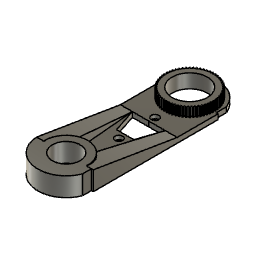
upperupperarm v1 (Autodesk Fusion 360 design; units mm, degrees)
Autodesk Fusion 360 part; units mm, degrees
sketch "lower_upper_sketch" plane through (0, 0, 0) normal (0, 0, 1) x (1, 0, 0)
  line L0 (-4.5, 9.5706) -> (-4.4999, -10)
  line L1 (0, 35.45) -> (-12.8784, 35.3615)
  circle A0 centre (0, 40.45) radius 1.75
  line L2 (0.0001, 16.7501) -> (-6.8648, 16.738)
  line L3 (0.0001, 16.7501) -> (6.9, 16.7501)
  line L4 (-4.4999, -10) -> (4.5001, -10)
  arc A1 (-4.7617, 10.2248) -> (4.7581, 10.2136) centre (0, 11.75) ccw
  arc A2 (-0.0001, 35.45) -> (0, 35.45) centre (0, 40.45) ccw
  line L5 (4.5001, -10) -> (4.5, 9.5706)
  circle A3 centre (0, 68.7017) radius 14
  line L6 (21.4115, 61.7879) -> (4.7581, 10.2136)
  circle A4 centre (0, 11.75) radius 1.75
  arc A5 (0, 45.45) -> (0, 45.45) centre (0, 67.95) ccw
  arc A6 (21.4115, 61.7879) -> (-21.4114, 61.7879) centre (0, 68.7017) ccw
  line L7 (-21.4114, 61.7879) -> (-4.7514, 10.193)
  line L8 (0, 35.45) -> (12.8942, 35.4107)
  line L9 (-4.7555, 10.2057) -> (-4.7555, 10.2055)
  circle A7 centre (50, 40.45) radius 1.75
  arc A8 (50, 45.45) -> (50.0001, 45.45) centre (50, 67.95) ccw
  circle A9 centre (50, 11.75) radius 1.75
  line L10 (50, 35.45) -> (36.9725, 35.45)
  arc A10 (72.5, 67.95) -> (29, 76.0277) centre (50, 67.95) ccw
  line L11 (50, 35.45) -> (63.0276, 35.45)
  circle A11 centre (50, 67.95) radius 14
  line L12 (50.0001, 16.7501) -> (43.1001, 16.7501)
  arc A12 (49.9999, 35.45) -> (50, 35.45) centre (50, 40.45) ccw
  line L13 (50.0001, 16.7501) -> (56.9, 16.7501)
  line L14 (50, 90.45) -> (50, -52.55) construction
  line L15 (27.5, 67.95) -> (27.5, -30.05)
  line L16 (72.5, 67.95) -> (72.5, -30.05)
  line L17 (63.0276, 35.45) -> (56.9, 16.7501)
  line L18 (36.9725, 35.45) -> (43.1001, 16.7501)
  circle A13 centre (50, -30.05) radius 11
  arc A14 (29, -38.1278) -> (72.5, -30.05) centre (50, -30.05) ccw
  line L19 (27.5, -30.05) -> (29, -30.05)
  line L20 (29, -30.05) -> (29, -38.1278)
  line L21 (27.5, 67.95) -> (29, 67.95)
  line L22 (29, 67.95) -> (29, 76.0277)
  line L23 (63.0276, 35.45) -> (72.5, 35.45)
  line L24 (36.9725, 35.45) -> (27.5, 35.45)
  circle A15 centre (50, -30.05) radius 17
  circle A16 centre (50, 11.75) radius 3
  circle A17 centre (50, 40.45) radius 3
  line L25 (58.5, -15.3276) -> (41.5, -15.3276)
  line L26 (63.0276, 35.45) -> (58.5, -15.3276)
  line L27 (36.9725, 35.45) -> (41.5, -15.3276)
  line L28 (50, 67.95) -> (69.5, 67.95)
  line L29 (69.5, 67.95) -> (69.5, 68.7)
  line L30 (69.5, 67.95) -> (69.5, 67.2)
  line L31 (69.5, 67.95) -> (68.5, 67.95)
  line L32 (68.5, 67.95) -> (68.5, 68.45)
  line L33 (68.5, 67.95) -> (68.5, 67.45)
  line L34 (68.5, 67.45) -> (69.5, 67.2)
  line L35 (69.5, 68.7) -> (68.5, 68.45)
  line L36 (68.4509, 69.3865) -> (69.4716, 69.2424)
  line L37 (68.3987, 69.8838) -> (68.4509, 69.3865)
  line L38 (68.3987, 69.8838) -> (68.3464, 70.381)
  line L39 (69.3148, 70.7342) -> (68.3464, 70.381)
  line L40 (68.1997, 71.3073) -> (69.2298, 71.2707)
  line L41 (68.0957, 71.7964) -> (68.1997, 71.3073)
  line L42 (68.0957, 71.7964) -> (67.9918, 72.2854)
  line L43 (68.918, 72.7379) -> (67.9918, 72.2854)
  line L44 (67.7491, 73.1913) -> (68.7774, 73.2625)
  line L45 (67.5946, 73.6668) -> (67.7491, 73.1913)
  line L46 (67.5946, 73.6668) -> (67.4401, 74.1423)
  line L47 (68.3139, 74.6891) -> (67.4401, 74.1423)
  line L48 (67.104, 75.0179) -> (68.1192, 75.1962)
  line L49 (66.9006, 75.4746) -> (67.104, 75.0179)
  line L50 (66.9006, 75.4746) -> (66.6972, 75.9314)
  line L51 (67.5091, 76.5665) -> (66.6972, 75.9314)
  line L52 (66.2715, 76.767) -> (67.2625, 77.0505)
  line L53 (66.0215, 77.2) -> (66.2715, 76.767)
  line L54 (66.0215, 77.2) -> (65.7715, 77.633)
  line L55 (66.5125, 78.3495) -> (65.7715, 77.633)
  line L56 (65.2607, 78.4195) -> (66.2167, 78.805)
  line L57 (64.9668, 78.824) -> (65.2607, 78.4195)
  line L58 (64.9668, 78.824) -> (64.6729, 79.2285)
  line L59 (65.335, 80.0186) -> (64.6729, 79.2285)
  line L60 (64.0828, 79.9573) -> (64.9932, 80.4407)
  line L61 (63.7482, 80.3289) -> (64.0828, 79.9573)
  line L62 (63.7482, 80.3289) -> (63.4136, 80.7005)
  line L63 (63.9895, 81.5554) -> (63.4136, 80.7005)
  line L64 (62.7505, 81.3636) -> (63.6054, 81.9395)
  line L65 (62.3789, 81.6982) -> (62.7505, 81.3636)
  line L66 (62.3789, 81.6982) -> (62.0074, 82.0327)
  line L67 (62.4907, 82.9432) -> (62.0074, 82.0327)
  line L68 (61.2785, 82.6229) -> (62.0686, 83.285)
  line L69 (60.874, 82.9168) -> (61.2785, 82.6229)
  line L70 (60.874, 82.9168) -> (60.4695, 83.2107)
  line L71 (60.8551, 84.1667) -> (60.4695, 83.2107)
  line L72 (59.683, 83.7215) -> (60.3995, 84.4625)
  line L73 (59.25, 83.9715) -> (59.683, 83.7215)
  line L74 (59.25, 83.9715) -> (58.817, 84.2215)
  line L75 (59.1005, 85.2125) -> (58.817, 84.2215)
  line L76 (57.9814, 84.6472) -> (58.6165, 85.4591)
  line L77 (57.5246, 84.8506) -> (57.9814, 84.6472)
  line L78 (57.5246, 84.8506) -> (57.0679, 85.054)
  line L79 (57.2462, 86.0692) -> (57.0679, 85.054)
  line L80 (56.1924, 85.39) -> (56.7391, 86.2638)
  line L81 (55.7168, 85.5445) -> (56.1924, 85.39)
  line L82 (55.7168, 85.5445) -> (55.2413, 85.699)
  line L83 (55.3126, 86.7274) -> (55.2413, 85.699)
  line L84 (54.3355, 85.9418) -> (54.7879, 86.8679)
  line L85 (53.8464, 86.0457) -> (54.3355, 85.9418)
  line L86 (53.8464, 86.0457) -> (53.3573, 86.1497)
  line L87 (53.3207, 87.1798) -> (53.3573, 86.1497)
  line L88 (52.4311, 86.2964) -> (52.7842, 87.2648)
  line L89 (51.9338, 86.3487) -> (52.4311, 86.2964)
  line L90 (51.9338, 86.3487) -> (51.4365, 86.4009)
  line L91 (51.2924, 87.4216) -> (51.4365, 86.4009)
  line L92 (50.5, 86.45) -> (50.75, 87.45)
  line L93 (50, 86.45) -> (50.5, 86.45)
  line L94 (50, 86.45) -> (49.5, 86.45)
  line L95 (49.25, 87.45) -> (49.5, 86.45)
  line L96 (48.5635, 86.4009) -> (48.7076, 87.4216)
  line L97 (48.0662, 86.3487) -> (48.5635, 86.4009)
  line L98 (48.0662, 86.3487) -> (47.569, 86.2964)
  line L99 (47.2158, 87.2648) -> (47.569, 86.2964)
  line L100 (46.6427, 86.1497) -> (46.6793, 87.1798)
  line L101 (46.1536, 86.0457) -> (46.6427, 86.1497)
  line L102 (46.1536, 86.0457) -> (45.6646, 85.9418)
  line L103 (45.2121, 86.8679) -> (45.6646, 85.9418)
  line L104 (44.7587, 85.699) -> (44.6875, 86.7274)
  line L105 (44.2832, 85.5445) -> (44.7587, 85.699)
  line L106 (44.2832, 85.5445) -> (43.8077, 85.39)
  line L107 (43.2609, 86.2638) -> (43.8077, 85.39)
  line L108 (42.9322, 85.054) -> (42.7538, 86.0692)
  line L109 (42.4754, 84.8506) -> (42.9322, 85.054)
  line L110 (42.4754, 84.8506) -> (42.0186, 84.6472)
  line L111 (41.3835, 85.4591) -> (42.0186, 84.6472)
  line L112 (41.183, 84.2215) -> (40.8995, 85.2125)
  line L113 (40.75, 83.9715) -> (41.183, 84.2215)
  line L114 (40.75, 83.9715) -> (40.317, 83.7215)
  line L115 (39.6005, 84.4625) -> (40.317, 83.7215)
  line L116 (39.5305, 83.2107) -> (39.145, 84.1667)
  line L117 (39.126, 82.9168) -> (39.5305, 83.2107)
  line L118 (39.126, 82.9168) -> (38.7215, 82.6229)
  line L119 (37.9314, 83.285) -> (38.7215, 82.6229)
  line L120 (37.9927, 82.0327) -> (37.5093, 82.9432)
  line L121 (37.6211, 81.6982) -> (37.9927, 82.0327)
  line L122 (37.6211, 81.6982) -> (37.2495, 81.3636)
  line L123 (36.3946, 81.9395) -> (37.2495, 81.3636)
  line L124 (36.5864, 80.7005) -> (36.0105, 81.5554)
  line L125 (36.2518, 80.3289) -> (36.5864, 80.7005)
  line L126 (36.2518, 80.3289) -> (35.9173, 79.9573)
  line L127 (35.0068, 80.4407) -> (35.9173, 79.9573)
  line L128 (35.3271, 79.2285) -> (34.665, 80.0186)
  line L129 (35.0332, 78.824) -> (35.3271, 79.2285)
  line L130 (35.0332, 78.824) -> (34.7393, 78.4195)
  line L131 (33.7833, 78.805) -> (34.7393, 78.4195)
  line L132 (34.2285, 77.633) -> (33.4875, 78.3495)
  line L133 (33.9785, 77.2) -> (34.2285, 77.633)
  line L134 (33.9785, 77.2) -> (33.7285, 76.767)
  line L135 (32.7375, 77.0505) -> (33.7285, 76.767)
  line L136 (33.3028, 75.9314) -> (32.4909, 76.5665)
  line L137 (33.0994, 75.4746) -> (33.3028, 75.9314)
  line L138 (33.0994, 75.4746) -> (32.8961, 75.0179)
  line L139 (31.8808, 75.1962) -> (32.8961, 75.0179)
  line L140 (32.56, 74.1423) -> (31.6862, 74.6891)
  line L141 (32.4055, 73.6668) -> (32.56, 74.1423)
  line L142 (32.4055, 73.6668) -> (32.251, 73.1913)
  line L143 (31.2226, 73.2625) -> (32.251, 73.1913)
  line L144 (32.0082, 72.2854) -> (31.0821, 72.7379)
  line L145 (31.9043, 71.7964) -> (32.0082, 72.2854)
  line L146 (31.9043, 71.7964) -> (31.8003, 71.3073)
  line L147 (30.7702, 71.2707) -> (31.8003, 71.3073)
  line L148 (31.6536, 70.381) -> (30.6852, 70.7342)
  line L149 (31.6014, 69.8838) -> (31.6536, 70.381)
  line L150 (31.6014, 69.8838) -> (31.5491, 69.3865)
  line L151 (30.5284, 69.2424) -> (31.5491, 69.3865)
  line L152 (31.5, 68.45) -> (30.5, 68.7)
  line L153 (31.5, 67.95) -> (31.5, 68.45)
  line L154 (31.5, 67.95) -> (31.5, 67.45)
  line L155 (30.5, 67.2) -> (31.5, 67.45)
  line L156 (31.5491, 66.5135) -> (30.5284, 66.6576)
  line L157 (31.6014, 66.0162) -> (31.5491, 66.5135)
  line L158 (31.6014, 66.0162) -> (31.6536, 65.519)
  line L159 (30.6852, 65.1658) -> (31.6536, 65.519)
  line L160 (31.8003, 64.5927) -> (30.7702, 64.6293)
  line L161 (31.9043, 64.1036) -> (31.8003, 64.5927)
  line L162 (31.9043, 64.1036) -> (32.0082, 63.6146)
  line L163 (31.0821, 63.1621) -> (32.0082, 63.6146)
  line L164 (32.251, 62.7087) -> (31.2226, 62.6375)
  line L165 (32.4055, 62.2332) -> (32.251, 62.7087)
  line L166 (32.4055, 62.2332) -> (32.56, 61.7577)
  line L167 (31.6862, 61.2109) -> (32.56, 61.7577)
  line L168 (32.8961, 60.8821) -> (31.8808, 60.7038)
  line L169 (33.0994, 60.4254) -> (32.8961, 60.8821)
  line L170 (33.0994, 60.4254) -> (33.3028, 59.9686)
  line L171 (32.4909, 59.3335) -> (33.3028, 59.9686)
  line L172 (33.7285, 59.133) -> (32.7375, 58.8495)
  line L173 (33.9785, 58.7) -> (33.7285, 59.133)
  line L174 (33.9785, 58.7) -> (34.2285, 58.267)
  line L175 (33.4875, 57.5505) -> (34.2285, 58.267)
  line L176 (34.7393, 57.4805) -> (33.7833, 57.0949)
  line L177 (35.0332, 57.076) -> (34.7393, 57.4805)
  line L178 (35.0332, 57.076) -> (35.3271, 56.6715)
  line L179 (34.665, 55.8814) -> (35.3271, 56.6715)
  line L180 (35.9173, 55.9427) -> (35.0068, 55.4593)
  line L181 (36.2518, 55.5711) -> (35.9173, 55.9427)
  line L182 (36.2518, 55.5711) -> (36.5864, 55.1995)
  line L183 (36.0105, 54.3446) -> (36.5864, 55.1995)
  line L184 (37.2495, 54.5364) -> (36.3946, 53.9605)
  line L185 (37.6211, 54.2018) -> (37.2495, 54.5364)
  line L186 (37.6211, 54.2018) -> (37.9927, 53.8673)
  line L187 (37.5093, 52.9568) -> (37.9927, 53.8673)
  line L188 (38.7215, 53.2771) -> (37.9314, 52.615)
  line L189 (39.126, 52.9832) -> (38.7215, 53.2771)
  line L190 (39.126, 52.9832) -> (39.5305, 52.6893)
  line L191 (39.145, 51.7333) -> (39.5305, 52.6893)
  line L192 (40.317, 52.1785) -> (39.6005, 51.4375)
  line L193 (40.75, 51.9285) -> (40.317, 52.1785)
  line L194 (40.75, 51.9285) -> (41.183, 51.6785)
  line L195 (40.8995, 50.6875) -> (41.183, 51.6785)
  line L196 (42.0186, 51.2528) -> (41.3835, 50.4409)
  line L197 (42.4754, 51.0494) -> (42.0186, 51.2528)
  line L198 (42.4754, 51.0494) -> (42.9322, 50.846)
  line L199 (42.7538, 49.8308) -> (42.9322, 50.846)
  line L200 (43.8077, 50.51) -> (43.2609, 49.6362)
  line L201 (44.2832, 50.3554) -> (43.8077, 50.51)
  line L202 (44.2832, 50.3554) -> (44.7587, 50.2009)
  line L203 (44.6875, 49.1726) -> (44.7587, 50.2009)
  line L204 (45.6646, 49.9582) -> (45.2121, 49.0321)
  line L205 (46.1536, 49.8543) -> (45.6646, 49.9582)
  line L206 (46.1536, 49.8543) -> (46.6427, 49.7503)
  line L207 (46.6793, 48.7202) -> (46.6427, 49.7503)
  line L208 (47.569, 49.6036) -> (47.2158, 48.6352)
  line L209 (48.0662, 49.5513) -> (47.569, 49.6036)
  line L210 (48.0662, 49.5513) -> (48.5635, 49.4991)
  line L211 (48.7076, 48.4784) -> (48.5635, 49.4991)
  line L212 (49.5, 49.45) -> (49.25, 48.45)
  line L213 (50, 49.45) -> (49.5, 49.45)
  line L214 (50, 49.45) -> (50.5, 49.45)
  line L215 (50.75, 48.45) -> (50.5, 49.45)
  line L216 (51.4365, 49.4991) -> (51.2924, 48.4784)
  line L217 (51.9338, 49.5513) -> (51.4365, 49.4991)
  line L218 (51.9338, 49.5513) -> (52.4311, 49.6036)
  line L219 (52.7842, 48.6352) -> (52.4311, 49.6036)
  line L220 (53.3573, 49.7503) -> (53.3207, 48.7202)
  line L221 (53.8464, 49.8543) -> (53.3573, 49.7503)
  line L222 (53.8464, 49.8543) -> (54.3355, 49.9582)
  line L223 (54.7879, 49.0321) -> (54.3355, 49.9582)
  line L224 (55.2413, 50.2009) -> (55.3126, 49.1726)
  line L225 (55.7168, 50.3554) -> (55.2413, 50.2009)
  line L226 (55.7168, 50.3554) -> (56.1924, 50.51)
  line L227 (56.7391, 49.6362) -> (56.1924, 50.51)
  line L228 (57.0679, 50.846) -> (57.2462, 49.8308)
  line L229 (57.5246, 51.0494) -> (57.0679, 50.846)
  line L230 (57.5246, 51.0494) -> (57.9814, 51.2528)
  line L231 (58.6165, 50.4409) -> (57.9814, 51.2528)
  line L232 (58.817, 51.6785) -> (59.1005, 50.6875)
  line L233 (59.25, 51.9285) -> (58.817, 51.6785)
  line L234 (59.25, 51.9285) -> (59.683, 52.1785)
  line L235 (60.3995, 51.4375) -> (59.683, 52.1785)
  line L236 (60.4695, 52.6893) -> (60.8551, 51.7333)
  line L237 (60.874, 52.9832) -> (60.4695, 52.6893)
  line L238 (60.874, 52.9832) -> (61.2785, 53.2771)
  line L239 (62.0686, 52.615) -> (61.2785, 53.2771)
  line L240 (62.0074, 53.8673) -> (62.4907, 52.9568)
  line L241 (62.3789, 54.2018) -> (62.0074, 53.8673)
  line L242 (62.3789, 54.2018) -> (62.7505, 54.5364)
  line L243 (63.6054, 53.9605) -> (62.7505, 54.5364)
  line L244 (63.4136, 55.1995) -> (63.9895, 54.3446)
  line L245 (63.7482, 55.5711) -> (63.4136, 55.1995)
  line L246 (63.7482, 55.5711) -> (64.0828, 55.9427)
  line L247 (64.9932, 55.4593) -> (64.0828, 55.9427)
  line L248 (64.6729, 56.6715) -> (65.335, 55.8814)
  line L249 (64.9668, 57.076) -> (64.6729, 56.6715)
  line L250 (64.9668, 57.076) -> (65.2607, 57.4805)
  line L251 (66.2167, 57.0949) -> (65.2607, 57.4805)
  line L252 (65.7715, 58.267) -> (66.5125, 57.5505)
  line L253 (66.0215, 58.7) -> (65.7715, 58.267)
  line L254 (66.0215, 58.7) -> (66.2715, 59.133)
  line L255 (67.2625, 58.8495) -> (66.2715, 59.133)
  line L256 (66.6972, 59.9686) -> (67.5091, 59.3335)
  line L257 (66.9006, 60.4254) -> (66.6972, 59.9686)
  line L258 (66.9006, 60.4254) -> (67.104, 60.8821)
  line L259 (68.1192, 60.7038) -> (67.104, 60.8821)
  line L260 (67.4401, 61.7577) -> (68.3139, 61.2109)
  line L261 (67.5946, 62.2332) -> (67.4401, 61.7577)
  line L262 (67.5946, 62.2332) -> (67.7491, 62.7087)
  line L263 (68.7774, 62.6375) -> (67.7491, 62.7087)
  line L264 (67.9918, 63.6146) -> (68.918, 63.1621)
  line L265 (68.0957, 64.1036) -> (67.9918, 63.6146)
  line L266 (68.0957, 64.1036) -> (68.1997, 64.5927)
  line L267 (69.2298, 64.6293) -> (68.1997, 64.5927)
  line L268 (68.3464, 65.519) -> (69.3148, 65.1658)
  line L269 (68.3987, 66.0162) -> (68.3464, 65.519)
  line L270 (68.3987, 66.0162) -> (68.4509, 66.5135)
  line L271 (69.4716, 66.6576) -> (68.4509, 66.5135)
  line L272 (29, -31.05) -> (33.0294, -31.05)
  line L273 (72.5, -31.05) -> (66.9706, -31.05)
  arc A18 (69.457, 66.6555) -> (69.4857, 67.2036) centre (50, 67.95) ccw
  arc A19 (69.4857, 68.6964) -> (69.457, 69.2445) centre (50, 67.95) ccw
  arc A20 (69.301, 70.7291) -> (69.2151, 71.2712) centre (50, 67.95) ccw
  arc A21 (68.9047, 72.7314) -> (68.7627, 73.2615) centre (50, 67.95) ccw
  arc A22 (68.3014, 74.6813) -> (68.1047, 75.1937) centre (50, 67.95) ccw
  arc A23 (67.4975, 76.5574) -> (67.2483, 77.0464) centre (50, 67.95) ccw
  arc A24 (66.5019, 78.3393) -> (66.203, 78.7995) centre (50, 67.95) ccw
  arc A25 (65.3255, 80.0073) -> (64.9802, 80.4338) centre (50, 67.95) ccw
  arc A26 (63.9813, 81.5432) -> (63.5932, 81.9312) centre (50, 67.95) ccw
  arc A27 (62.4838, 82.9302) -> (62.0573, 83.2755) centre (50, 67.95) ccw
  arc A28 (60.8496, 84.153) -> (60.3893, 84.4519) centre (50, 67.95) ccw
  arc A29 (59.0964, 85.1983) -> (58.6075, 85.4475) centre (50, 67.95) ccw
  arc A30 (57.2437, 86.0547) -> (56.7313, 86.2513) centre (50, 67.95) ccw
  arc A31 (55.3115, 86.7127) -> (54.7814, 86.8547) centre (50, 67.95) ccw
  arc A32 (53.3212, 87.1651) -> (52.7792, 87.2509) centre (50, 67.95) ccw
  arc A33 (51.2945, 87.407) -> (50.7464, 87.4357) centre (50, 67.95) ccw
  arc A34 (49.2536, 87.4357) -> (48.7055, 87.407) centre (50, 67.95) ccw
  arc A35 (47.2209, 87.2509) -> (46.6788, 87.1651) centre (50, 67.95) ccw
  arc A36 (45.2186, 86.8547) -> (44.6885, 86.7127) centre (50, 67.95) ccw
  arc A37 (43.2687, 86.2513) -> (42.7564, 86.0547) centre (50, 67.95) ccw
  arc A38 (41.3926, 85.4475) -> (40.9036, 85.1983) centre (50, 67.95) ccw
  arc A39 (39.6107, 84.4519) -> (39.1505, 84.153) centre (50, 67.95) ccw
  arc A40 (37.9427, 83.2755) -> (37.5162, 82.9302) centre (50, 67.95) ccw
  arc A41 (36.4068, 81.9312) -> (36.0188, 81.5432) centre (50, 67.95) ccw
  arc A42 (35.0199, 80.4338) -> (34.6745, 80.0073) centre (50, 67.95) ccw
  arc A43 (33.797, 78.7995) -> (33.4981, 78.3393) centre (50, 67.95) ccw
  arc A44 (32.7517, 77.0464) -> (32.5025, 76.5574) centre (50, 67.95) ccw
  arc A45 (31.8953, 75.1937) -> (31.6987, 74.6813) centre (50, 67.95) ccw
  arc A46 (31.2373, 73.2615) -> (31.0953, 72.7314) centre (50, 67.95) ccw
  arc A47 (30.7849, 71.2712) -> (30.6991, 70.7291) centre (50, 67.95) ccw
  arc A48 (30.543, 69.2445) -> (30.5143, 68.6964) centre (50, 67.95) ccw
  arc A49 (30.5143, 67.2036) -> (30.543, 66.6555) centre (50, 67.95) ccw
  arc A50 (30.6991, 65.1708) -> (30.7849, 64.6288) centre (50, 67.95) ccw
  arc A51 (31.0953, 63.1686) -> (31.2373, 62.6385) centre (50, 67.95) ccw
  arc A52 (31.6987, 61.2187) -> (31.8953, 60.7063) centre (50, 67.95) ccw
  arc A53 (32.5025, 59.3425) -> (32.7517, 58.8536) centre (50, 67.95) ccw
  arc A54 (33.4981, 57.5607) -> (33.797, 57.1005) centre (50, 67.95) ccw
  arc A55 (34.6745, 55.8927) -> (35.0199, 55.4662) centre (50, 67.95) ccw
  arc A56 (36.0188, 54.3568) -> (36.4068, 53.9687) centre (50, 67.95) ccw
  arc A57 (37.5162, 52.9698) -> (37.9427, 52.6245) centre (50, 67.95) ccw
  arc A58 (39.1505, 51.747) -> (39.6107, 51.4481) centre (50, 67.95) ccw
  arc A59 (40.9036, 50.7017) -> (41.3926, 50.4525) centre (50, 67.95) ccw
  arc A60 (42.7564, 49.8453) -> (43.2687, 49.6486) centre (50, 67.95) ccw
  arc A61 (44.6885, 49.1873) -> (45.2186, 49.0453) centre (50, 67.95) ccw
  arc A62 (46.6788, 48.7349) -> (47.2209, 48.6491) centre (50, 67.95) ccw
  arc A63 (48.7055, 48.493) -> (49.2536, 48.4643) centre (50, 67.95) ccw
  arc A64 (50.7464, 48.4643) -> (51.2945, 48.493) centre (50, 67.95) ccw
  arc A65 (52.7792, 48.6491) -> (53.3212, 48.7349) centre (50, 67.95) ccw
  arc A66 (54.7814, 49.0453) -> (55.3115, 49.1873) centre (50, 67.95) ccw
  arc A67 (56.7313, 49.6486) -> (57.2437, 49.8453) centre (50, 67.95) ccw
  arc A68 (58.6075, 50.4525) -> (59.0964, 50.7017) centre (50, 67.95) ccw
  arc A69 (60.3893, 51.4481) -> (60.8496, 51.747) centre (50, 67.95) ccw
  arc A70 (62.0573, 52.6245) -> (62.4838, 52.9698) centre (50, 67.95) ccw
  arc A71 (63.5932, 53.9687) -> (63.9813, 54.3568) centre (50, 67.95) ccw
  arc A72 (64.9802, 55.4662) -> (65.3255, 55.8927) centre (50, 67.95) ccw
  arc A73 (66.203, 57.1005) -> (66.5019, 57.5607) centre (50, 67.95) ccw
  arc A74 (67.2483, 58.8536) -> (67.4975, 59.3425) centre (50, 67.95) ccw
  arc A75 (68.1047, 60.7063) -> (68.3014, 61.2187) centre (50, 67.95) ccw
  arc A76 (68.7627, 62.6385) -> (68.9047, 63.1686) centre (50, 67.95) ccw
  arc A77 (69.2151, 64.6288) -> (69.301, 65.1708) centre (50, 67.95) ccw
  dimension "d1" = 22.5
  dimension "d2" = 28.2517
  dimension "d3" = 143
  dimension "d4" = 45
  dimension "d5" = 98
  dimension "d6" = 22
  dimension "d7" = 1.5
  dimension "d8" = 1.5
  dimension "d10" = 34
  dimension "d11" = 6
  dimension "d12" = 6
  dimension "d13" = 17
  dimension "d14" = 39
  dimension "d15" = 0.75
  dimension "d16" = 0.75
  dimension "d17" = 1
  dimension "d18" = 0.5
  dimension "d19" = 0.5
  dimension "d21" = 360
  dimension "d22" = 1
  dimension "d23" = 1
  constraint coincident L7 L2.end
  constraint tangent A1 L7
  constraint coincident L7 L9.start
  constraint coincident A1 L9.end
  constraint coincident L7 L1.end
  constraint coincident L6 L8.end
  constraint tangent A6 L7
  constraint tangent L6 A6
  constraint tangent A1 L6
  constraint concentric A3 A6
  constraint perpendicular L11 L14
  constraint coincident L14 A13.centre
  constraint tangent L15 A14
  constraint tangent L16 A14
  constraint concentric A13 A14
  constraint coincident A10 L14.start
  constraint perpendicular L14 L19
  constraint perpendicular L19 L20
  constraint perpendicular L15 L21
  constraint perpendicular L21 L22
  constraint coincident L16 L23.end
  constraint perpendicular L16 L23
  constraint coincident L15 L24.end
  constraint perpendicular L15 L24
  constraint concentric A13 A15
  constraint concentric A9 A16
  constraint concentric A7 A17
  constraint coincident A15 L25.start
  constraint coincident A15 L25.end
  constraint perpendicular L14 L25
  constraint concentric A8 A18
  constraint coincident A8.centre A10.centre
  constraint coincident L28.end A18
  constraint perpendicular L14 L28
  constraint perpendicular L28 L29
  constraint perpendicular L28 L30
  constraint perpendicular L30 L31
  constraint perpendicular L28 L32
  constraint perpendicular L28 L33
  constraint coincident A15 L272.end
  constraint perpendicular L20 L272
  constraint coincident A15 L273.end
  constraint perpendicular L16 L273
  constraint coincident L271 A18.start
  constraint coincident L34 A18.end
  measures "d1" radius of A6
  measures "d2" distance of A0.centre A3.centre
  measures "d3" distance of L14.start L14.end
  measures "d4" diameter of A14
  measures "d5" vertical distance of A8.centre A13.centre
  measures "d6" diameter of A13
  measures "d7" distance of L15.end L19.end
  measures "d8" distance of L15.start L21.end
  measures "d10" diameter of A15
  measures "d11" diameter of A16
  measures "d12" diameter of A17
  measures "d13" distance of L25.start L25.end
  measures "d14" diameter of A18
  measures "d15" distance of L28.end L29.end
  measures "d16" distance of L28.end L30.end
  measures "d17" distance of L28.end L31.end
  measures "d18" distance of L31.end L32.end
  measures "d19" distance of L31.end L33.end
  measures "d22" distance of L19.end L272.start
  measures "d23" distance of L16.end L273.start
extrude "Extrude2" add sketch "lower_upper_sketch" against normal blind 4 contours A8 A10 L21 L22 | A8 L11 A12 L16 L23 | A8 L10 A12 L15 L24 | A12 | L12 L13 L17 L18 A15 L26 L27 | L28 L29 L31 L32 L35 | L28 L30 L31 L33 L34 makes body 1
sketch "Sketch2" plane through (27.5, 0, 0) normal (-1, 0, 0) x (0, -1, 0)
  line L0 (-35.45, 0) -> (-67.95, 0)
  line L1 (-67.95, 0) -> (-67.95, -4)
  line L2 (-67.95, -4) -> (-35.45, -4)
  line L3 (-35.45, -4) -> (-35.45, 0)
  line L4 (-35.45, -4) -> (-35.45, 0)
  line L5 (-35.45, 0) -> (31.05, 0)
  line L6 (31.05, 0) -> (-35.45, 0)
  line L7 (31.05, 0) -> (31.05, -15)
  line L8 (31.05, -15) -> (-35.45, -15)
  line L9 (-35.45, -15) -> (-35.45, -4)
  line L10 (-35.45, -4) -> (31.05, -15)
  constraint coincident L2.end L3.start
  constraint coincident L0.start L3.end
  constraint perpendicular L4 L5
  constraint perpendicular L6 L7
  constraint perpendicular L7 L8
  constraint perpendicular L2 L9
extrude "Extrude5" add sketch "Sketch2" against normal blind 45 contours L3 L4 L5 L6 L7 L10 bodies 1
extrude "Extrude6" add sketch "lower_upper_sketch" against normal blind 15 contours A14 L20 A15 L272 L273 | A15 L25 | A15 L25 bodies 1
extrude "Extrude3" add sketch "lower_upper_sketch" against normal blind 1 separate body contours A16 | A17 makes body 2 at (52.9963, 11.6005, -0.6667) makes body 3 at (52.9963, 40.3005, -0.6667)
extrude "Extrude4" add sketch "lower_upper_sketch" against normal blind 11 separate body contours L32 L33 L34 L35 L36 L37 L38 L39 L40 L41 L42 L43 L44 L45 L46 L47 L48 L49 L50 L51 L52 L53 L54 L55 L56 L57 L58 L59 L60 L61 L62 L63 L64 L65 L66 L67 L68 L69 L70 L71 L72 L73 L74 L75 L76 L77 L78 L79 L80 L81 L82 L83 L84 L85 L86 L87 L88 L89 L90 L91 L92 L93 L94 L95 L96 L97 L98 L99 L100 L101 L102 L103 L104 L105 L106 L107 L108 L109 L110 L111 L112 L113 L114 L115 L116 L117 L118 L119 L120 L121 L122 L123 L124 L125 L126 L127 L128 L129 L130 L131 L132 L133 L134 L135 L136 L137 L138 L139 L140 L141 L142 L143 L144 L145 L146 L147 L148 L149 L150 L151 L152 L153 L154 L155 L156 L157 L158 L159 L160 L161 L162 L163 L164 L165 L166 L167 L168 L169 L170 L171 L172 L173 L174 L175 L176 L177 L178 L179 L180 L181 L182 L183 L184 L185 L186 L187 L188 L189 L190 L191 L192 L193 L194 L195 L196 L197 L198 L199 L200 L201 L202 L203 L204 L205 L206 L207 L208 L209 L210 L211 L212 L213 L214 L215 L216 L217 L218 L219 L220 L221 L222 L223 L224 L225 L226 L227 L228 L229 L230 L231 L232 L233 L234 L235 L236 L237 L238 L239 L240 L241 L242 L243 L244 L245 L246 L247 L248 L249 L250 L251 L252 L253 L254 L255 L256 L257 L258 L259 L260 L261 L262 L263 L264 L265 L266 L267 L268 L269 L270 L271 A18 A19 A20 A21 A22 A23 A24 A25 A26 A27 A28 A29 A30 A31 A32 A33 A34 A35 A36 A37 A38 A39 A40 A41 A42 A43 A44 A45 A46 A47 A48 A49 A50 A51 A52 A53 A54 A55 A56 A57 A58 A59 A60 A61 A62 A63 A64 A65 A66 A67 A68 A69 A70 A71 A72 A73 A74 A75 A76 A77 makes body 4
extrude "Extrude7" cut sketch "lower_upper_sketch" against normal blind 55 contours A7 | L10 L11 L12 L13 L17 L18 | L12 L13 L17 L18 A15 L26 L27 | A9 | A13 | A16 | A17 bodies 1 2 3
extrude "Extrude8" add sketch "lower_upper_sketch" against normal blind 4 contours L12 L13 L17 L18 A15 L26 L27 bodies 1 2 3
extrude "Extrude9" add sketch "lower_upper_sketch" against normal blind 1 separate body contours A16 | A17 makes body 5 at (52.9963, 11.6005, -0.6667) makes body 6 at (52.9963, 40.3005, -0.6667)
copy_body "Body->Comp1" bodies 6 removing the originals makes body 7 in component "Component"
copy_body "CutPasteBodies1" bodies 1 removing the originals makes body 8 in component "Component"
copy_body "CutPasteBodies2" bodies 4 removing the originals makes body 9 in component "Component"
copy_body "CutPasteBodies3" bodies 5 removing the originals makes body 10 in component "Component"
component "Component" placed x (1, 0, 0) y (0, 1, 0) z (0, 0, 1) at (0, 0, 0)
